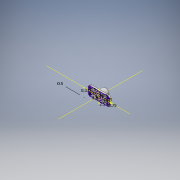
# Autodesk Inventor part: 7b
Saved by Autodesk Inventor 2018 (Build 220112000, 112)
## iProperties
Created: 2018-10-23
Part Number: 7b
Material: Generic
Document SubType Name: Modeling
Designer: Jerry
Density: 1 g/cm^3
Appearance: Default
Author: Jerry
Autodesk Inventor part; units mm, degrees
ref_plane "YZ Plane" through (0, 0, 0) normal (1, 0, 0) x (0, 1, 0)
ref_plane "XZ Plane" through (0, 0, 0) normal (0, 1, 0) x (-1, 0, 0)
sketch "Sketch1" plane through (0, 0, 0) normal (0, 1, 0) x (-1, 0, 0)
  line L0 (2.5, -1.25) -> (-2.5, -1.25)
  line L1 (-3, -0.75) -> (-3, 0.75)
  line L2 (-2.5, 1.25) -> (2.5, 1.25)
  line L3 (3, 0.75) -> (3, -0.75)
  arc A0 (2.5, -1.25) -> (3, -0.75) centre (2.5, -0.75) ccw
  arc A1 (-3, -0.75) -> (-2.5, -1.25) centre (-2.5, -0.75) ccw
  arc A2 (-2.5, 1.25) -> (-3, 0.75) centre (-2.5, 0.75) ccw
  arc A3 (3, 0.75) -> (2.5, 1.25) centre (2.5, 0.75) ccw
  circle A4 centre (2.5, -0.75) radius 0.25
  circle A5 centre (-2.5, -0.75) radius 0.25
  circle A6 centre (-2.5, 0.75) radius 0.25
  circle A7 centre (2.5, 0.75) radius 0.25
  circle A8 centre (0, 0) radius 1
  circle A9 centre (0, 0) radius 0.625
  line L4 (0, -1.895) -> (0, 1.895) projected
  line L5 (4.345, 0) -> (-4.345, 0) projected
  line L6 (3, -0.1875) -> (0.9823, -0.1875)
  line L7 (3, 0.1875) -> (0.9823, 0.1875)
  line L8 (-3, -0.1875) -> (-0.9823, -0.1875)
  line L9 (-3, 0.1875) -> (-0.9823, 0.1875)
  point P0 (-2.5, 0.75)
  dimension "d9" = 2
  dimension "d0" = 0.75
  dimension "d1" = 0.75
  dimension "d2" = 2.5
  dimension "d3" = 2.5
  dimension "d4" = 0.5
  dimension "d5" = 0.5
  dimension "d6" = 0.5
  dimension "d7" = 0.5
  dimension "d8" = 0.5
  dimension "d10" = 1.25
  dimension "d11" = 0.375
  constraints: 16 end point, 9 centre point, 9 coincident, 8 point on circle, 8 tangent, 6 symmetric about line, 3 equal radius, 3 parallel, 2 horizontal alignment, 2 vertical alignment, 1 horizontal, 1 perpendicular, 1 point on line, 3 other
  measures "d0" vertical distance of point (0, 0) point (-2.5, -0.75)
  measures "d1" vertical distance of point (0, 0) point (-2.5, 0.75)
  measures "d2" horizontal distance of point (0, 0) point (-2.5, -0.75)
  measures "d3" horizontal distance of point (0, 0) point (2.5, -0.75)
  measures "d4" radius of A0
  measures "d5" diameter of A4
  measures "d6" diameter of A5
  measures "d7" diameter of A6
  measures "d8" diameter of A7
  measures "d10" diameter of A9
  measures "d11" distance between parallel lines of L7 L6
extrude "Extrusion1" add sketch "Sketch1" along normal blind 0.5 contours L0 L4 A8 L6 L3 A0 | L0 A1 L1 L8 A8 L4 | L6 A8 L5 L3 | L8 L1 L5 A8 | L5 A8 L7 L3 | L5 L1 L9 A8 | L7 A8 L4 L2 A3 L3 | L9 L1 A2 L2 L4 A8
extrude "Extrusion2" add sketch "Sketch1" along normal blind 2 contours L4 A9 L5 A8 | A8 L5 A9 L4 | A8 L4 A9 L5 | L5 A9 L4 A8
sketch "Sketch2" plane through (0, 0.5, 0) normal (0, 1, 0) x (1, 0, 0)
  circle A0 centre (0, 0) radius 1 projected
  line L0 (3, -0.75) -> (3, 0.75) projected
  line L1 (-3, 0.75) -> (-3, -0.75) projected
  line L2 (-3, 0.1875) -> (-0.9823, 0.1875) projected
  line L3 (-3, -0.1875) -> (-0.9823, -0.1875) projected
  line L4 (3, -0.1875) -> (0.9823, -0.1875) projected
  line L5 (3, 0.1875) -> (0.9823, 0.1875) projected
ref_plane "Work Plane1" through (-3, 0.5, 0.1875) normal (0, 0, 1) x (1, 0, 0)
sketch "Sketch3" plane through (-3, 0.5, 0.1875) normal (0, 0, 1) x (1, 0, 0)
  line L0 (0, -0.5) -> (0, 0) projected
  line L1 (2.0177, 1.25) -> (2.0177, 0) projected
  line L2 (0, 0) -> (2.0177, 1.25)
  line L3 (4, 1.25) -> (3.9823, 1.25) projected
  line L4 (6, -0.5) -> (6, 0) projected
  line L5 (3.9823, 1.25) -> (6, 0)
  line L6 (0, 0) -> (2.0177, 0)
  line L7 (2.0177, 1.25) -> (2.0177, 0)
  line L8 (3.9823, 1.25) -> (3.9823, 0) projected
  line L9 (6, 0) -> (3.9823, 0) projected
  line L10 (3.9823, 1.25) -> (3.9823, 0)
  line L11 (6, 0) -> (6, 1.25) projected
  line L12 (3.9823, 0) -> (6, 0)
  point P0 (3, -0.5)
  constraints: 12 end point, 3 perpendicular, 1 horizontal
extrude "Extrusion4" add sketch "Sketch3" against normal blind 0.375
body "Solid1"
